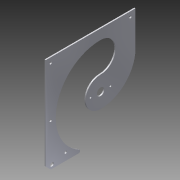
# Autodesk Inventor part: rail gearbox mounting
Saved by Autodesk Inventor 2015 (Build 190159000, 159)
## iProperties
Created: 2015-02-22
Part Number: rail gearbox mounting
Material: Aluminum 6061
Document SubType Name: Modeling
Designer: Jarod
Density: 2.7 g/cm^3
Appearance: Aluminum - Flat
Author: Jarod
Autodesk Inventor part; units mm, degrees
ref_plane "YZ Plane" through (0, 0, 0) normal (1, 0, 0) x (0, 1, 0)
ref_plane "XZ Plane" through (0, 0, 0) normal (0, 1, 0) x (-1, 0, 0)
ref_plane "XY Plane" through (0, 0, 0) normal (0, 0, 1) x (1, 0, 0)
sketch "Sketch1" plane through (0, 0, 0) normal (1, 0, 0) x (0, 1, 0)
  circle A0 centre (0, 0) radius 50.8 construction
  circle A1 centre (82.55, 0) radius 31.75 construction
  circle A2 centre (-82.55, 0) radius 31.75 construction
  circle A3 centre (0, 0) radius 114.3 construction
  circle A4 centre (0, 0) radius 38.1 construction
  arc A5 (38.1, 0) -> (114.3, 0) centre (76.2, 0) ccw construction
  arc A6 (-38.1, 0) -> (139.7, 0) centre (50.8, 0) ccw construction
  line L0 (50.8, -88.9) -> (139.7, -88.9) construction
  line L1 (139.7, -88.9) -> (139.7, 0) construction
  line L2 (139.7, 0) -> (-114.3, 0) construction
  line L3 (-114.3, 0) -> (-114.3, 139.7) construction
  line L4 (-114.3, 139.7) -> (139.7, 139.7) construction
  line L5 (139.7, 139.7) -> (139.7, 0) construction
  arc A7 (10.165, 139.7) -> (-114.3, 80.9625) centre (0, 0) ccw construction
  line L6 (-114.3, 139.7) -> (-114.3, 38.1) construction
  line L7 (-114.3, 38.1) -> (-107.7631, 38.1) construction
  arc A8 (-10.165, 139.7) -> (-114.3, 80.9625) centre (0, 0) ccw
  line L8 (-10.165, 139.7) -> (139.7, 139.7)
  line L9 (139.7, 139.7) -> (139.7, -88.9)
  line L10 (139.7, -88.9) -> (50.8, -88.9)
  arc A9 (-38.1, 0) -> (50.8, -88.9) centre (50.8, 0) ccw
  arc A10 (38.1, 0) -> (-38.1, 0) centre (0, 0) ccw
  arc A11 (38.1, 0) -> (114.3, 0) centre (76.2, 0) ccw
  arc A12 (114.3, 0) -> (-107.7631, 38.1) centre (0, 0) ccw
  line L11 (-107.7631, 38.1) -> (-114.3, 38.1)
  line L12 (-114.3, 80.9625) -> (-114.3, 38.1)
  dimension "d1" = 63.5
  dimension "d0" = 101.6
  dimension "d2" = 63.5
  dimension "d3" = 82.55
  dimension "d4" = 82.55
  dimension "d5" = 0
  dimension "d6" = 0
  dimension "d7" = 228.6
  dimension "d8" = 76.2
  dimension "d9" = 76.2
  dimension "d10" = 177.8
  dimension "d11" = 88.9
  dimension "d12" = 139.7
  dimension "d13" = 0
  dimension "d14" = 254
  dimension "d15" = 139.7
  dimension "d16" = 0
  dimension "d17" = 58.7375
  dimension "d18" = 101.6
  constraints: 26 end point, 22 point on circle, 12 centre point, 4 coincident, 4 tangent, 3 collinear, 3 horizontal, 3 perpendicular, 3 point on line, 2 concentric, 2 parallel, 1 horizontal alignment, 2 other
  measures "d0" diameter of A0
  measures "d2" diameter of A2
  measures "d3" distance of point (0, 0) A2.centre
  measures "d4" distance of point (0, 0) point (82.55, 0)
  measures "d5" vertical distance of point (0, 0) A2.centre
  measures "d6" vertical distance of point (0, 0) point (82.55, 0)
  measures "d7" diameter of A3
  measures "d8" diameter of A4
  measures "d9" distance of A4.start A3.start
  measures "d10" distance of A4.end L1.end
  measures "d11" radius of A6
  measures "d12" distance of point (0, 0) L1.end
  measures "d13" vertical distance of point (0, 0) L1.end
  measures "d14" distance of L3.end L4.end
  measures "d15" distance of L2.end L3.end
  measures "d16" distance from line of L3 L12.start
  measures "d17" distance from line of L4 L12.start
  measures "d18" distance of L3.end L6.end
extrude "Extrusion1" add sketch "Sketch1" along normal blind 3.175
sketch "Sketch2" plane through (3.175, 0, 0) normal (1, 0, 0) x (0, 0, -1)
  arc A0 (0, 38.1) -> (0, -38.1) centre (0, 0) ccw projected
  arc A1 (0, -38.1) -> (88.9, 50.8) centre (0, 50.8) ccw projected
  line L0 (88.9, 50.8) -> (88.9, 139.7) projected
  line L1 (88.9, 139.7) -> (-139.7, 139.7) projected
  line L2 (-139.7, 139.7) -> (-139.7, -10.165) projected
  arc A2 (-139.7, -10.165) -> (-80.9625, -114.3) centre (0, 0) ccw projected
  line L3 (-80.9625, -114.3) -> (-38.1, -114.3) projected
  line L4 (-38.1, -114.3) -> (-38.1, -107.7631) projected
  arc A3 (0, 114.3) -> (-38.1, -107.7631) centre (0, 0) ccw projected
  arc A4 (0, 38.1) -> (0, 114.3) centre (0, 76.2) ccw projected
  line L5 (-38.1, -114.3) -> (-114.3, -114.3)
  line L6 (-114.3, -114.3) -> (-114.3, -107.95)
  line L7 (-114.3, -107.95) -> (-38.1, -107.95)
  line L8 (-38.1, -107.95) -> (-38.1, -114.3)
  arc A5 (0, 114.3) -> (-38.1, -107.7631) centre (0, 0) ccw projected
  line L9 (-38.1, -114.3) -> (-52.3634, -114.3)
  line L10 (-52.3634, -114.3) -> (-52.3634, -101.6)
  line L11 (-52.3634, -101.6) -> (-38.1, -101.6)
  line L12 (-38.1, -101.6) -> (-38.1, -114.3)
  point P0 (0, 0)
  dimension "d24" = 76.2
  dimension "d25" = 6.35
  dimension "d26" = 12.7
  constraints: 16 end point, 4 parallel, 2 horizontal, 2 perpendicular, 1 point on circle
  measures "d24" distance of L6.end L7.end
  measures "d25" distance of L5.end L6.end
  measures "d26" distance of L9.end L10.end
extrude "Extrusion2" cut sketch "Sketch2" against normal blind 3.175 contours L11 L12 A3 | A3 L4 L7 L10 | L10 L3 A2 L7 | L7 L4 L3 L10 | A2 L5 L6 L7
sketch "Sketch3" plane through (3.175, 0, 0) normal (1, 0, 0) x (0, 0, -1)
  line L0 (-89.2536, -107.95) -> (-52.3634, -107.95) projected
  line L1 (-52.3634, -107.95) -> (-52.3634, -101.6) projected
  arc A0 (0, 114.3) -> (-52.3634, -101.6) centre (0, 0) ccw projected
  arc A1 (0, 38.1) -> (0, 114.3) centre (0, 76.2) ccw projected
  arc A2 (0, 38.1) -> (0, -38.1) centre (0, 0) ccw projected
  arc A3 (0, -38.1) -> (88.9, 50.8) centre (0, 50.8) ccw projected
  line L2 (88.9, 50.8) -> (88.9, 139.7) projected
  line L3 (88.9, 139.7) -> (-139.7, 139.7) projected
  line L4 (-139.7, 139.7) -> (-139.7, -10.165) projected
  arc A4 (-139.7, -10.165) -> (-89.2536, -107.95) centre (0, 0) ccw projected
  point P0 (0, 0)
  point P1 (-127, 127)
  point P2 (76.2, 127)
  point P3 (-88.9, -88.9)
  point P4 (-127, 0)
  dimension "d29" = 12.7
  dimension "d30" = 12.7
  dimension "d31" = 12.7
  dimension "d32" = 12.7
  dimension "d33" = 12.7
  dimension "d34" = 139.7
  dimension "d35" = 88.9
  dimension "d36" = 88.9
  measures "d29" distance from line of L3 point (-127, 127)
  measures "d30" distance from line of point (-127, 127) L4
  measures "d31" distance from line of L3 point (76.2, 127)
  measures "d32" distance from line of L2 point (76.2, 127)
  measures "d33" distance from line of L4 point (-127, 0)
  measures "d34" distance from line of L3 point (-127, 0)
  measures "d35" horizontal distance of A0.centre point (-88.9, -88.9)
  measures "d36" horizontal distance of A4.centre point (-88.9, -88.9)
hole "Hole1" at (3.175, 127, 127) at (3.175, 127, -76.2) at (3.175, -88.9, 88.9) at (3.175, 0, 127) direction (-1, 0, 0) diameter 6.35 end through all
sketch "Sketch4" plane through (3.175, 0, 0) normal (1, 0, 0) x (0, 0, -1)
  circle A0 centre (-88.9, -88.9) radius 3.175 projected
  circle A1 centre (-127, 127) radius 3.175 projected
  circle A2 centre (76.2, 127) radius 3.175 projected
  circle A3 centre (-127, 0) radius 3.175 projected
  line L0 (-89.2536, -107.95) -> (-52.3634, -107.95) projected
  line L1 (-52.3634, -107.95) -> (-52.3634, -101.6) projected
  arc A4 (0, 114.3) -> (-52.3634, -101.6) centre (0, 0) ccw projected
  arc A5 (0, 38.1) -> (0, 114.3) centre (0, 76.2) ccw projected
  arc A6 (0, 38.1) -> (0, -38.1) centre (0, 0) ccw projected
  arc A7 (0, -38.1) -> (88.9, 50.8) centre (0, 50.8) ccw projected
  line L2 (88.9, 50.8) -> (88.9, 139.7) projected
  line L3 (88.9, 139.7) -> (-139.7, 139.7) projected
  line L4 (-139.7, 139.7) -> (-139.7, -10.165) projected
  arc A8 (-139.7, -10.165) -> (-89.2536, -107.95) centre (0, 0) ccw projected
  circle A9 centre (0, 0) radius 9.525
  circle A10 centre (-25.4, 0) radius 2.3813
  circle A11 centre (25.4, 0) radius 2.3813
  point P0 (0, 0)
  dimension "d44" = 0
  dimension "d45" = 0
  dimension "d46" = 25.4
  dimension "d47" = 25.4
  dimension "d55" = 19.05
  dimension "d56" = 4.7625
  dimension "d57" = 4.7625
  constraints: 3 centre point, 3 coincident
  measures "d44" vertical distance of point (0, 0) point (-25.4, 0)
  measures "d45" vertical distance of A8.centre point (25.4, 0)
  measures "d46" distance of A4.centre point (25.4, 0)
  measures "d47" distance of point (0, 0) point (-25.4, 0)
  measures "d55" diameter of A9
  measures "d56" diameter of A10
  measures "d57" diameter of A11
extrude "Extrusion3" cut sketch "Sketch4" against normal blind 3.175 contours A9 | A10 | A11
sketch "Sketch5" plane through (3.175, 0, 0) normal (1, 0, 0) x (0, 0, -1)
  circle A0 centre (25.4, 0) radius 2.3813 projected
  circle A1 centre (-25.4, 0) radius 2.3813 projected
  circle A2 centre (0, 0) radius 9.525 projected
  circle A3 centre (-88.9, -88.9) radius 3.175 projected
  circle A4 centre (-127, 127) radius 3.175 projected
  circle A5 centre (76.2, 127) radius 3.175 projected
  circle A6 centre (-127, 0) radius 3.175 projected
  line L0 (-89.2536, -107.95) -> (-52.3634, -107.95) projected
  line L1 (-52.3634, -107.95) -> (-52.3634, -101.6) projected
  arc A7 (0, 114.3) -> (-52.3634, -101.6) centre (0, 0) ccw projected
  arc A8 (0, 38.1) -> (0, 114.3) centre (0, 76.2) ccw projected
  arc A9 (0, 38.1) -> (0, -38.1) centre (0, 0) ccw projected
  arc A10 (0, -38.1) -> (88.9, 50.8) centre (0, 50.8) ccw projected
  line L2 (88.9, 50.8) -> (88.9, 139.7) projected
  line L3 (88.9, 139.7) -> (-139.7, 139.7) projected
  line L4 (-139.7, 139.7) -> (-139.7, -10.165) projected
  arc A11 (-139.7, -10.165) -> (-89.2536, -107.95) centre (0, 0) ccw projected
  line L5 (-139.7, -10.165) -> (-139.7, -107.95) construction
  line L6 (-139.7, -107.95) -> (-89.2536, -107.95) construction
  line L7 (-139.7, -107.95) -> (-127, -107.95) construction
  line L8 (-127, -107.95) -> (-127, -95.25) construction
  line L9 (-127, -95.25) -> (-139.7, -95.25) construction
  line L10 (-139.7, -95.25) -> (-139.7, -107.95) construction
  line L11 (-139.7, -10.165) -> (-139.7, -95.25)
  line L12 (-139.7, -95.25) -> (-127, -107.95)
  line L13 (-127, -107.95) -> (-89.2536, -107.95)
  point P0 (0, 0)
  dimension "d60" = 12.7
  dimension "d61" = 12.7
  constraints: 18 end point, 3 perpendicular, 2 parallel, 1 collinear, 1 horizontal, 1 vertical
  measures "d60" distance of L9.end L8.end
  measures "d61" distance of L8.end L7.end
extrude "Extrusion4" add sketch "Sketch5" against normal blind 3.175 contours L13 L12 L11 A11
sketch "Sketch6" plane through (3.175, 0, 0) normal (1, 0, 0) x (0, 0, -1)
  circle A0 centre (25.4, 0) radius 2.3813 projected
  circle A1 centre (-25.4, 0) radius 2.3813 projected
  circle A2 centre (0, 0) radius 9.525 projected
  circle A3 centre (-88.9, -88.9) radius 3.175 projected
  circle A4 centre (-127, 127) radius 3.175 projected
  circle A5 centre (76.2, 127) radius 3.175 projected
  circle A6 centre (-127, 0) radius 3.175 projected
  line L0 (-127, -107.95) -> (-52.3634, -107.95) projected
  line L1 (-52.3634, -107.95) -> (-52.3634, -101.6) projected
  arc A7 (0, 114.3) -> (-52.3634, -101.6) centre (0, 0) ccw projected
  arc A8 (0, 38.1) -> (0, 114.3) centre (0, 76.2) ccw projected
  arc A9 (0, 38.1) -> (0, -38.1) centre (0, 0) ccw projected
  arc A10 (0, -38.1) -> (88.9, 50.8) centre (0, 50.8) ccw projected
  line L2 (88.9, 50.8) -> (88.9, 139.7) projected
  line L3 (88.9, 139.7) -> (-139.7, 139.7) projected
  line L4 (-139.7, 139.7) -> (-139.7, -95.25) projected
  line L5 (-139.7, -95.25) -> (-127, -107.95) projected
  point P0 (0, 0)
  point P1 (-123.825, -98.425)
  dimension "d64" = 15.875
  dimension "d65" = 9.525
  measures "d64" distance from line of L4 point (-123.825, -98.425)
  measures "d65" distance from line of L0 point (-123.825, -98.425)
hole "Hole3" at (3.175, -98.425, 123.825) direction (-1, 0, 0) diameter 9.525 end through all
fillet "Fillet1" radius 3.175 2 edges at (1.5875, -107.95, 52.3634) (1.5875, -101.6, 52.3634)
body "Solid1"
